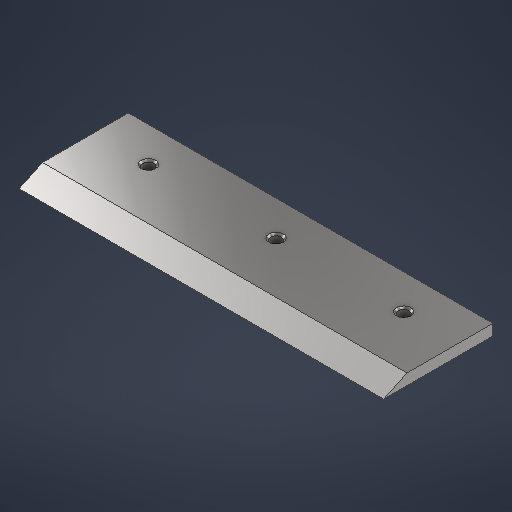
# Autodesk Inventor part: Knife
Saved by Autodesk Inventor 2026.2 (Build 302298010, 298A)
## iProperties
Created: 2026-04-01
Part Number: Knife
Material: Ocel, uhlík
Document SubType Name: Modeling
Designer: zak
Density: 7.85 g/cm^3
Appearance: Pololeštěná
Author: zak
Autodesk Inventor part; units mm, degrees
ref_plane "YZ Plane" through (0, 0, 0) normal (1, 0, 0) x (0, 1, 0)
ref_plane "XZ Plane" through (0, 0, 0) normal (0, 1, 0) x (-1, 0, 0)
ref_plane "XY Plane" through (0, 0, 0) normal (0, 0, 1) x (1, 0, 0)
sketch "Náčrt1" plane through (0, 0, 0) normal (1, 0, 0) x (0, 1, 0)
  line L0 (1.5, 15) -> (-1.5, 15)
  line L1 (-1.5, 15) -> (-1.5, -15)
  line L2 (-1.5, -15) -> (1.5, -15)
  line L3 (1.5, -15) -> (1.5, 15)
  line L4 (1.5, 15) -> (-1.5, -15) construction
  line L5 (-1.5, 15) -> (1.5, -15) construction
  line L6 (-1.5, 15) -> (1.5, 8.5665)
  point P0 (0, 0)
  dimension "d0" = 3
  dimension "d1" = 30
  dimension "d2" = 25
  constraints: 14 end point, 2 midpoint, 2 parallel, 1 horizontal, 1 perpendicular, 1 point on line
  measures "d0" distance between parallel lines of L1 L3
  measures "d1" distance between parallel lines of L0 L2
  measures "d2" angle of L1 L6
extrude "Vysunutí1" add sketch "Náčrt1" along normal mid plane 100 contours L6 L3 L2 L1
sketch "Náčrt2" plane through (-50, -1.5, -15) normal (0, -1, 0) x (1, 0, 0)
  circle A0 centre (85, 9.5) radius 1.5
  circle A1 centre (50, 9.5) radius 1.5
  circle A2 centre (15, 9.5) radius 1.5
  line L0 (0, 0) -> (100, 0) projected
  line L1 (100, 30) -> (100, 0) projected
  line L2 (0, 30) -> (100, 30) projected
  line L3 (0, 0) -> (0, 30) projected
  line L4 (100, 9.5) -> (0, 9.5) construction
  line L5 (50, 0) -> (50, 30) construction
  point P0 (50, 15)
  point P1 (50, 9.5)
  dimension "d5" = 9.5
  dimension "d6" = 3
  dimension "d7" = 35
  dimension "d8" = 3
  constraints: 4 end point, 4 point on line, 3 centre point, 3 midpoint, 1 coincident, 1 perpendicular, 1 other
  measures "d5" distance between parallel lines of L0 L4
  measures "d6" diameter of A1
  measures "d7" distance of A1.centre A2.centre
  measures "d8" diameter of A2
extrude "Vysunutí2" cut sketch "Náčrt2" against normal through all contours A0 | A1 | A2
thread "Závit1" size "M3x0.5" class "6H" standard "ANSI Metric M Profile" full length
thread "Závit2" size "M3x0.5" class "6H" standard "ANSI Metric M Profile" full length
thread "Závit3" size "M3x0.5" class "6H" standard "ANSI Metric M Profile" full length
sketch "Náčrt3" plane through (-50, -1.5, -15) normal (0, -1, 0) x (1, 0, 0)
  circle A0 centre (15, 9.5) radius 1.5 projected
  circle A1 centre (50, 9.5) radius 1.5 projected
  circle A2 centre (85, 9.5) radius 1.5 projected
  line L0 (0, 0) -> (100, 0) projected
  line L1 (100, 30) -> (100, 0) projected
  line L2 (0, 30) -> (100, 30) projected
  line L3 (0, 0) -> (0, 30) projected
  line L4 (99.3391, 0.6963) -> (54.869, 0.6963) construction
  line L5 (54.869, 0.6963) -> (54.869, 9.6594) construction
  line L6 (54.869, 9.6594) -> (99.3391, 9.6594) construction
  line L7 (99.3391, 9.6594) -> (99.3391, 0.6963) construction
  line L8 (98.3181, 1.9686) -> (98.5044, 1.9686)
  line L9 (98.5044, 1.9686) -> (99.0575, 0.8908)
  line L10 (99.0575, 0.8908) -> (99.0575, 1.9686)
  line L11 (99.0575, 1.9686) -> (99.2125, 1.9686)
  line L12 (99.2125, 1.9686) -> (99.2125, 0.7186)
  line L13 (99.2125, 0.7186) -> (98.9765, 0.7186)
  line L14 (98.9765, 0.7186) -> (98.473, 1.7083)
  line L15 (98.473, 1.7083) -> (98.473, 0.7186)
  line L16 (98.473, 0.7186) -> (98.3181, 0.7186)
  line L17 (98.3181, 0.7186) -> (98.3181, 1.9686)
  spline S0 degree 2 poles (97.6698, 1.9899) (97.8946, 1.9899) (98.1418, 1.7376) (98.1418, 1.5046) knots 0 0 0 1 2 2 2
  spline S1 degree 2 poles (98.1418, 1.5046) (98.1418, 1.2757) (97.9017, 1.0042) (97.7083, 1.0042) knots 0 0 0 1 2 2 2
  spline S2 degree 2 poles (97.7083, 1.0042) (97.6211, 1.0042) (97.4864, 1.0549) (97.4368, 1.1086) knots 0 0 0 1 2 2 2
  spline S3 degree 2 poles (97.4368, 1.1086) (97.3861, 1.1623) (97.3324, 1.3172) (97.3324, 1.4297) knots 0 0 0 1 2 2 2
  line L18 (97.3324, 1.4297) -> (97.3324, 1.5158)
  line L19 (97.3324, 1.5158) -> (97.9818, 1.5158)
  spline S4 degree 2 poles (97.9818, 1.5158) (97.9818, 1.6789) (97.8177, 1.8521) (97.6718, 1.8521) knots 0 0 0 1 2 2 2
  spline S5 degree 2 poles (97.6718, 1.8521) (97.6201, 1.8521) (97.5198, 1.8288) (97.4793, 1.8106) knots 0 0 0 1 2 2 2
  spline S6 degree 2 poles (97.4793, 1.8106) (97.4368, 1.7903) (97.378, 1.7548) (97.3588, 1.7386) knots 0 0 0 1 2 2 2
  line L20 (97.3588, 1.7386) -> (97.3497, 1.7386)
  line L21 (97.3497, 1.7386) -> (97.3497, 1.9108)
  spline S7 degree 2 poles (97.3497, 1.9108) (97.377, 1.922) (97.4601, 1.9544) (97.4925, 1.9635) knots 0 0 0 1 2 2 2
  spline S8 degree 2 poles (97.4925, 1.9635) (97.5381, 1.9767) (97.613, 1.9899) (97.6698, 1.9899) knots 0 0 0 1 2 2 2
  spline S9 degree 2 poles (97.4864, 1.3952) (97.4884, 1.3314) (97.5148, 1.2382) (97.5401, 1.2068) knots 0 0 0 1 2 2 2
  spline S10 degree 2 poles (97.5401, 1.2068) (97.5674, 1.1714) (97.6536, 1.1339) (97.7174, 1.1339) knots 0 0 0 1 2 2 2
  spline S11 degree 2 poles (97.7174, 1.1339) (97.7802, 1.1339) (97.8683, 1.1714) (97.9048, 1.2078) knots 0 0 0 1 2 2 2
  spline S12 degree 2 poles (97.9048, 1.2078) (97.9402, 1.2453) (97.9767, 1.3355) (97.9818, 1.3952) knots 0 0 0 1 2 2 2
  line L22 (97.9818, 1.3952) -> (97.4864, 1.3952)
  spline S13 degree 2 poles (96.4015, 1.4996) (96.4015, 1.7366) (96.6294, 1.9949) (96.8199, 1.9949) knots 0 0 0 1 2 2 2
  spline S14 degree 2 poles (96.8199, 1.9949) (97.0154, 1.9949) (97.2392, 1.7285) (97.2392, 1.4996) knots 0 0 0 1 2 2 2
  spline S15 degree 2 poles (97.2392, 1.4996) (97.2392, 1.2646) (97.0083, 1.0042) (96.8199, 1.0042) knots 0 0 0 1 2 2 2
  spline S16 degree 2 poles (96.8199, 1.0042) (96.6294, 1.0042) (96.4015, 1.2636) (96.4015, 1.4996) knots 0 0 0 1 2 2 2
  spline S17 degree 2 poles (96.5646, 1.4996) (96.5646, 1.3172) (96.6973, 1.14) (96.8199, 1.14) knots 0 0 0 1 2 2 2
  spline S18 degree 2 poles (96.8199, 1.14) (96.9424, 1.14) (97.0762, 1.3172) (97.0762, 1.4996) knots 0 0 0 1 2 2 2
  spline S19 degree 2 poles (97.0762, 1.4996) (97.0762, 1.6768) (96.9424, 1.8592) (96.8199, 1.8592) knots 0 0 0 1 2 2 2
  spline S20 degree 2 poles (96.8199, 1.8592) (96.6983, 1.8592) (96.5646, 1.6799) (96.5646, 1.4996) knots 0 0 0 1 2 2 2
  spline S21 degree 2 poles (95.8788, 1.9909) (96.0146, 1.9909) (96.205, 1.9341) (96.2891, 1.8936) knots 0 0 0 1 2 2 2
  line L23 (96.2891, 1.8936) -> (96.2891, 1.685)
  line L24 (96.2891, 1.685) -> (96.2769, 1.685)
  spline S22 degree 2 poles (96.2769, 1.685) (96.1949, 1.7619) (95.9872, 1.847) (95.891, 1.847) knots 0 0 0 1 2 2 2
  spline S23 degree 2 poles (95.891, 1.847) (95.7532, 1.847) (95.6124, 1.7326) (95.6124, 1.6384) knots 0 0 0 1 2 2 2
  spline S24 degree 2 poles (95.6124, 1.6384) (95.6124, 1.5634) (95.6864, 1.4702) (95.7664, 1.4469) knots 0 0 0 1 2 2 2
  spline S25 degree 2 poles (95.7664, 1.4469) (95.8241, 1.4307) (95.9204, 1.4084) (95.9923, 1.3902) knots 0 0 0 1 2 2 2
  spline S26 degree 2 poles (95.9923, 1.3902) (96.0571, 1.373) (96.1594, 1.3213) (96.1989, 1.2798) knots 0 0 0 1 2 2 2
  spline S27 degree 2 poles (96.1989, 1.2798) (96.2374, 1.2382) (96.28, 1.1268) (96.28, 1.0539) knots 0 0 0 1 2 2 2
  spline S28 degree 2 poles (96.28, 1.0539) (96.28, 0.9019) (96.0429, 0.6963) (95.8596, 0.6963) knots 0 0 0 1 2 2 2
  spline S29 degree 2 poles (95.8596, 0.6963) (95.7542, 0.6963) (95.5679, 0.7378) (95.4878, 0.7773) knots 0 0 0 1 2 2 2
  line L25 (95.4878, 0.7773) -> (95.4878, 0.9759)
  line L26 (95.4878, 0.9759) -> (95.5, 0.9759)
  spline S30 degree 2 poles (95.5, 0.9759) (95.5598, 0.9212) (95.7461, 0.8401) (95.8484, 0.8401) knots 0 0 0 1 2 2 2
  spline S31 degree 2 poles (95.8484, 0.8401) (95.9639, 0.8401) (96.1068, 0.9485) (96.1068, 1.0367) knots 0 0 0 1 2 2 2
  spline S32 degree 2 poles (96.1068, 1.0367) (96.1068, 1.1157) (96.0227, 1.2099) (95.9437, 1.2311) knots 0 0 0 1 2 2 2
  spline S33 degree 2 poles (95.9437, 1.2311) (95.891, 1.2453) (95.738, 1.2818) (95.6874, 1.297) knots 0 0 0 1 2 2 2
  spline S34 degree 2 poles (95.6874, 1.297) (95.5587, 1.3365) (95.4392, 1.4955) (95.4392, 1.612) knots 0 0 0 1 2 2 2
  spline S35 degree 2 poles (95.4392, 1.612) (95.4392, 1.686) (95.499, 1.8278) (95.5527, 1.8774) knots 0 0 0 1 2 2 2
  spline S36 degree 2 poles (95.5527, 1.8774) (95.6124, 1.9321) (95.7644, 1.9909) (95.8788, 1.9909) knots 0 0 0 1 2 2 2
  line L27 (94.5529, 1.9686) -> (94.7109, 1.9686)
  line L28 (94.7109, 1.9686) -> (94.7109, 1.8653)
  spline S37 degree 2 poles (94.7109, 1.8653) (94.7838, 1.9291) (94.9145, 1.9949) (94.9955, 1.9949) knots 0 0 0 1 2 2 2
  spline S38 degree 2 poles (94.9955, 1.9949) (95.0563, 1.9949) (95.1647, 1.9544) (95.2042, 1.9108) knots 0 0 0 1 2 2 2
  spline S39 degree 2 poles (95.2042, 1.9108) (95.2447, 1.8673) (95.2893, 1.7346) (95.2893, 1.6394) knots 0 0 0 1 2 2 2
  line L29 (95.2893, 1.6394) -> (95.2893, 1.0306)
  line L30 (95.2893, 1.0306) -> (95.1313, 1.0306)
  line L31 (95.1313, 1.0306) -> (95.1313, 1.5654)
  spline S40 degree 2 poles (95.1313, 1.5654) (95.1313, 1.6404) (95.1201, 1.7386) (95.1009, 1.7751) knots 0 0 0 1 2 2 2
  spline S41 degree 2 poles (95.1009, 1.7751) (95.0816, 1.8116) (95.0158, 1.845) (94.954, 1.845) knots 0 0 0 1 2 2 2
  spline S42 degree 2 poles (94.954, 1.845) (94.8963, 1.845) (94.7656, 1.7792) (94.7109, 1.7315) knots 0 0 0 1 2 2 2
  line L32 (94.7109, 1.7315) -> (94.7109, 1.0306)
  line L33 (94.7109, 1.0306) -> (94.5529, 1.0306)
  line L34 (94.5529, 1.0306) -> (94.5529, 1.9686)
  line L35 (93.2603, 1.9686) -> (93.2603, 1.4256)
  spline S43 degree 2 poles (93.2603, 1.4256) (93.2603, 1.3608) (93.2704, 1.2504) (93.2867, 1.22) knots 0 0 0 1 2 2 2
  spline S44 degree 2 poles (93.2867, 1.22) (93.3029, 1.1866) (93.3647, 1.1542) (93.4183, 1.1542) knots 0 0 0 1 2 2 2
  spline S45 degree 2 poles (93.4183, 1.1542) (93.467, 1.1542) (93.5784, 1.2139) (93.6371, 1.2707) knots 0 0 0 1 2 2 2
  spline S46 degree 2 poles (93.6371, 1.2707) (93.6361, 1.2848) (93.6341, 1.3243) (93.6341, 1.3507) knots 0 0 0 1 2 2 2
  line L36 (93.6341, 1.3507) -> (93.6341, 1.9686)
  line L37 (93.6341, 1.9686) -> (93.7921, 1.9686)
  line L38 (93.7921, 1.9686) -> (93.7921, 1.4256)
  spline S47 degree 2 poles (93.7921, 1.4256) (93.7921, 1.3608) (93.8023, 1.2504) (93.8185, 1.22) knots 0 0 0 1 2 2 2
  spline S48 degree 2 poles (93.8185, 1.22) (93.8347, 1.1866) (93.8965, 1.1542) (93.9501, 1.1542) knots 0 0 0 1 2 2 2
  spline S49 degree 2 poles (93.9501, 1.1542) (94.0008, 1.1542) (94.1132, 1.218) (94.1659, 1.2676) knots 0 0 0 1 2 2 2
  line L39 (94.1659, 1.2676) -> (94.1659, 1.9686)
  line L40 (94.1659, 1.9686) -> (94.3239, 1.9686)
  line L41 (94.3239, 1.9686) -> (94.3239, 1.0306)
  line L42 (94.3239, 1.0306) -> (94.1659, 1.0306)
  line L43 (94.1659, 1.0306) -> (94.1659, 1.1339)
  spline S50 degree 2 poles (94.1659, 1.1339) (94.1041, 1.0721) (93.9826, 1.0042) (93.9096, 1.0042) knots 0 0 0 1 2 2 2
  spline S51 degree 2 poles (93.9096, 1.0042) (93.8266, 1.0042) (93.6979, 1.0802) (93.6645, 1.1663) knots 0 0 0 1 2 2 2
  spline S52 degree 2 poles (93.6645, 1.1663) (93.5926, 1.0863) (93.4568, 1.0042) (93.3778, 1.0042) knots 0 0 0 1 2 2 2
  spline S53 degree 2 poles (93.3778, 1.0042) (93.317, 1.0042) (93.2178, 1.0417) (93.1813, 1.0843) knots 0 0 0 1 2 2 2
  spline S54 degree 2 poles (93.1813, 1.0843) (93.1438, 1.1268) (93.1023, 1.2544) (93.1023, 1.3507) knots 0 0 0 1 2 2 2
  line L44 (93.1023, 1.3507) -> (93.1023, 1.9686)
  line L45 (93.1023, 1.9686) -> (93.2603, 1.9686)
  spline S55 degree 2 poles (92.4732, 1.9899) (92.6981, 1.9899) (92.9453, 1.7376) (92.9453, 1.5046) knots 0 0 0 1 2 2 2
  spline S56 degree 2 poles (92.9453, 1.5046) (92.9453, 1.2757) (92.7052, 1.0042) (92.5117, 1.0042) knots 0 0 0 1 2 2 2
  spline S57 degree 2 poles (92.5117, 1.0042) (92.4246, 1.0042) (92.2899, 1.0549) (92.2403, 1.1086) knots 0 0 0 1 2 2 2
  spline S58 degree 2 poles (92.2403, 1.1086) (92.1896, 1.1623) (92.1359, 1.3172) (92.1359, 1.4297) knots 0 0 0 1 2 2 2
  line L46 (92.1359, 1.4297) -> (92.1359, 1.5158)
  line L47 (92.1359, 1.5158) -> (92.7852, 1.5158)
  spline S59 degree 2 poles (92.7852, 1.5158) (92.7852, 1.6789) (92.6211, 1.8521) (92.4753, 1.8521) knots 0 0 0 1 2 2 2
  spline S60 degree 2 poles (92.4753, 1.8521) (92.4236, 1.8521) (92.3233, 1.8288) (92.2828, 1.8106) knots 0 0 0 1 2 2 2
  spline S61 degree 2 poles (92.2828, 1.8106) (92.2403, 1.7903) (92.1815, 1.7548) (92.1623, 1.7386) knots 0 0 0 1 2 2 2
  line L48 (92.1623, 1.7386) -> (92.1531, 1.7386)
  line L49 (92.1531, 1.7386) -> (92.1531, 1.9108)
  spline S62 degree 2 poles (92.1531, 1.9108) (92.1805, 1.922) (92.2636, 1.9544) (92.296, 1.9635) knots 0 0 0 1 2 2 2
  spline S63 degree 2 poles (92.296, 1.9635) (92.3416, 1.9767) (92.4165, 1.9899) (92.4732, 1.9899) knots 0 0 0 1 2 2 2
  spline S64 degree 2 poles (92.2899, 1.3952) (92.2919, 1.3314) (92.3183, 1.2382) (92.3436, 1.2068) knots 0 0 0 1 2 2 2
  spline S65 degree 2 poles (92.3436, 1.2068) (92.3709, 1.1714) (92.457, 1.1339) (92.5209, 1.1339) knots 0 0 0 1 2 2 2
  spline S66 degree 2 poles (92.5209, 1.1339) (92.5837, 1.1339) (92.6718, 1.1714) (92.7083, 1.2078) knots 0 0 0 1 2 2 2
  spline S67 degree 2 poles (92.7083, 1.2078) (92.7437, 1.2453) (92.7802, 1.3355) (92.7852, 1.3952) knots 0 0 0 1 2 2 2
  line L50 (92.7852, 1.3952) -> (92.2899, 1.3952)
  spline S68 degree 2 poles (91.6031, 1.9899) (91.7004, 1.9899) (91.8614, 1.9301) (91.9192, 1.8693) knots 0 0 0 1 2 2 2
  spline S69 degree 2 poles (91.9192, 1.8693) (91.9769, 1.8095) (92.0407, 1.6252) (92.0407, 1.5016) knots 0 0 0 1 2 2 2
  spline S70 degree 2 poles (92.0407, 1.5016) (92.0407, 1.378) (91.9749, 1.1977) (91.9192, 1.1369) knots 0 0 0 1 2 2 2
  spline S71 degree 2 poles (91.9192, 1.1369) (91.8634, 1.0751) (91.6983, 1.0093) (91.6031, 1.0093) knots 0 0 0 1 2 2 2
  spline S72 degree 2 poles (91.6031, 1.0093) (91.5261, 1.0093) (91.3823, 1.0529) (91.3266, 1.0812) knots 0 0 0 1 2 2 2
  line L51 (91.3266, 1.0812) -> (91.3266, 1.2585)
  line L52 (91.3266, 1.2585) -> (91.3357, 1.2585)
  spline S73 degree 2 poles (91.3357, 1.2585) (91.3529, 1.2443) (91.4056, 1.2078) (91.4431, 1.1886) knots 0 0 0 1 2 2 2
  spline S74 degree 2 poles (91.4431, 1.1886) (91.4765, 1.1724) (91.5656, 1.1471) (91.6061, 1.1471) knots 0 0 0 1 2 2 2
  spline S75 degree 2 poles (91.6061, 1.1471) (91.7287, 1.1471) (91.8776, 1.3324) (91.8776, 1.5016) knots 0 0 0 1 2 2 2
  spline S76 degree 2 poles (91.8776, 1.5016) (91.8776, 1.6667) (91.7338, 1.8521) (91.6061, 1.8521) knots 0 0 0 1 2 2 2
  spline S77 degree 2 poles (91.6061, 1.8521) (91.5292, 1.8521) (91.3894, 1.7883) (91.3357, 1.7386) knots 0 0 0 1 2 2 2
  line L53 (91.3357, 1.7386) -> (91.3266, 1.7386)
  line L54 (91.3266, 1.7386) -> (91.3266, 1.9159)
  spline S78 degree 2 poles (91.3266, 1.9159) (91.3499, 1.9271) (91.4208, 1.9585) (91.4491, 1.9655) knots 0 0 0 1 2 2 2
  spline S79 degree 2 poles (91.4491, 1.9655) (91.4897, 1.9777) (91.5535, 1.9899) (91.6031, 1.9899) knots 0 0 0 1 2 2 2
  line L55 (98.1408, 4.0267) -> (98.3069, 4.0267)
  line L56 (98.3069, 4.0267) -> (98.3069, 2.9499)
  line L57 (98.3069, 2.9499) -> (98.6331, 3.6823)
  line L58 (98.6331, 3.6823) -> (98.7344, 3.6823)
  line L59 (98.7344, 3.6823) -> (99.0575, 2.9499)
  line L60 (99.0575, 2.9499) -> (99.0575, 4.0267)
  line L61 (99.0575, 4.0267) -> (99.2125, 4.0267)
  line L62 (99.2125, 4.0267) -> (99.2125, 2.7767)
  line L63 (99.2125, 2.7767) -> (98.9856, 2.7767)
  line L64 (98.9856, 2.7767) -> (98.6736, 3.4726)
  line L65 (98.6736, 3.4726) -> (98.3717, 2.7767)
  line L66 (98.3717, 2.7767) -> (98.1408, 2.7767)
  line L67 (98.1408, 2.7767) -> (98.1408, 4.0267)
  spline S80 degree 2 poles (97.377, 3.9274) (97.3963, 3.9416) (97.4611, 3.9922) (97.4915, 4.0074) knots 0 0 0 1 2 2 2
  spline S81 degree 2 poles (97.4915, 4.0074) (97.533, 4.0297) (97.611, 4.053) (97.6819, 4.053) knots 0 0 0 1 2 2 2
  spline S82 degree 2 poles (97.6819, 4.053) (97.7397, 4.053) (97.844, 4.0095) (97.8835, 3.9699) knots 0 0 0 1 2 2 2
  spline S83 degree 2 poles (97.8835, 3.9699) (97.921, 3.9315) (97.9666, 3.818) (97.9666, 3.7552) knots 0 0 0 1 2 2 2
  spline S84 degree 2 poles (97.9666, 3.7552) (97.9666, 3.658) (97.8845, 3.5202) (97.7954, 3.4807) knots 0 0 0 1 2 2 2
  spline S85 degree 2 poles (97.7954, 3.4807) (97.7164, 3.4442) (97.5016, 3.4169) (97.377, 3.4098) knots 0 0 0 1 2 2 2
  line L68 (97.377, 3.4098) -> (97.377, 3.3794)
  spline S86 degree 2 poles (97.377, 3.3794) (97.377, 3.3247) (97.4104, 3.2568) (97.4408, 3.2376) knots 0 0 0 1 2 2 2
  spline S87 degree 2 poles (97.4408, 3.2376) (97.4712, 3.2183) (97.5583, 3.2062) (97.6049, 3.2062) knots 0 0 0 1 2 2 2
  spline S88 degree 2 poles (97.6049, 3.2062) (97.6596, 3.2062) (97.8075, 3.2386) (97.8815, 3.27) knots 0 0 0 1 2 2 2
  line L69 (97.8815, 3.27) -> (97.8906, 3.27)
  line L70 (97.8906, 3.27) -> (97.8906, 3.1089)
  spline S89 degree 2 poles (97.8906, 3.1089) (97.847, 3.0968) (97.6839, 3.0664) (97.6039, 3.0664) knots 0 0 0 1 2 2 2
  spline S90 degree 2 poles (97.6039, 3.0664) (97.5067, 3.0664) (97.374, 3.0968) (97.3213, 3.1363) knots 0 0 0 1 2 2 2
  spline S91 degree 2 poles (97.3213, 3.1363) (97.2696, 3.1748) (97.219, 3.2973) (97.219, 3.3855) knots 0 0 0 1 2 2 2
  line L71 (97.219, 3.3855) -> (97.219, 4.0267)
  line L72 (97.219, 4.0267) -> (97.377, 4.0267)
  line L73 (97.377, 4.0267) -> (97.377, 3.9274)
  line L74 (97.377, 3.7957) -> (97.377, 3.5354)
  spline S92 degree 2 poles (97.377, 3.5354) (97.4337, 3.5405) (97.6049, 3.5577) (97.6586, 3.5739) knots 0 0 0 1 2 2 2
  spline S93 degree 2 poles (97.6586, 3.5739) (97.7214, 3.5931) (97.8035, 3.6732) (97.8035, 3.7441) knots 0 0 0 1 2 2 2
  spline S94 degree 2 poles (97.8035, 3.7441) (97.8035, 3.8251) (97.7123, 3.9071) (97.6252, 3.9071) knots 0 0 0 1 2 2 2
  spline S95 degree 2 poles (97.6252, 3.9071) (97.5512, 3.9071) (97.4297, 3.8433) (97.377, 3.7957) knots 0 0 0 1 2 2 2
  line L75 (96.2759, 4.0267) -> (96.4339, 4.0267)
  line L76 (96.4339, 4.0267) -> (96.4339, 3.9315)
  spline S96 degree 2 poles (96.4339, 3.9315) (96.4704, 3.9618) (96.5241, 4.0024) (96.5606, 4.0196) knots 0 0 0 1 2 2 2
  spline S97 degree 2 poles (96.5606, 4.0196) (96.594, 4.0358) (96.6659, 4.053) (96.7135, 4.053) knots 0 0 0 1 2 2 2
  spline S98 degree 2 poles (96.7135, 4.053) (96.7905, 4.053) (96.9202, 3.9892) (96.9657, 3.9274) knots 0 0 0 1 2 2 2
  spline S99 degree 2 poles (96.9657, 3.9274) (97.0113, 3.8656) (97.062, 3.6833) (97.062, 3.5648) knots 0 0 0 1 2 2 2
  spline S100 degree 2 poles (97.062, 3.5648) (97.062, 3.4412) (96.9982, 3.2609) (96.9424, 3.193) knots 0 0 0 1 2 2 2
  spline S101 degree 2 poles (96.9424, 3.193) (96.8908, 3.1322) (96.7459, 3.0623) (96.6659, 3.0623) knots 0 0 0 1 2 2 2
  spline S102 degree 2 poles (96.6659, 3.0623) (96.596, 3.0623) (96.4917, 3.0937) (96.4339, 3.1261) knots 0 0 0 1 2 2 2
  line L77 (96.4339, 3.1261) -> (96.4339, 2.721)
  line L78 (96.4339, 2.721) -> (96.2759, 2.721)
  line L79 (96.2759, 2.721) -> (96.2759, 4.0267)
  line L80 (96.4339, 3.7988) -> (96.4339, 3.2568)
  spline S103 degree 2 poles (96.4339, 3.2568) (96.4927, 3.2285) (96.5859, 3.2072) (96.6396, 3.2072) knots 0 0 0 1 2 2 2
  spline S104 degree 2 poles (96.6396, 3.2072) (96.7611, 3.2072) (96.8989, 3.3895) (96.8989, 3.5617) knots 0 0 0 1 2 2 2
  spline S105 degree 2 poles (96.8989, 3.5617) (96.8989, 3.7279) (96.7935, 3.9031) (96.6771, 3.9031) knots 0 0 0 1 2 2 2
  spline S106 degree 2 poles (96.6771, 3.9031) (96.6153, 3.9031) (96.4897, 3.8464) (96.4339, 3.7988) knots 0 0 0 1 2 2 2
  spline S107 degree 2 poles (95.6398, 4.0479) (95.8647, 4.0479) (96.1118, 3.7957) (96.1118, 3.5627) knots 0 0 0 1 2 2 2
  spline S108 degree 2 poles (96.1118, 3.5627) (96.1118, 3.3338) (95.8717, 3.0623) (95.6783, 3.0623) knots 0 0 0 1 2 2 2
  spline S109 degree 2 poles (95.6783, 3.0623) (95.5912, 3.0623) (95.4564, 3.113) (95.4068, 3.1667) knots 0 0 0 1 2 2 2
  spline S110 degree 2 poles (95.4068, 3.1667) (95.3561, 3.2204) (95.3025, 3.3753) (95.3025, 3.4878) knots 0 0 0 1 2 2 2
  line L81 (95.3025, 3.4878) -> (95.3025, 3.5739)
  line L82 (95.3025, 3.5739) -> (95.9518, 3.5739)
  spline S111 degree 2 poles (95.9518, 3.5739) (95.9518, 3.737) (95.7877, 3.9102) (95.6418, 3.9102) knots 0 0 0 1 2 2 2
  spline S112 degree 2 poles (95.6418, 3.9102) (95.5901, 3.9102) (95.4899, 3.8869) (95.4493, 3.8687) knots 0 0 0 1 2 2 2
  spline S113 degree 2 poles (95.4493, 3.8687) (95.4068, 3.8484) (95.348, 3.8129) (95.3288, 3.7967) knots 0 0 0 1 2 2 2
  line L83 (95.3288, 3.7967) -> (95.3197, 3.7967)
  line L84 (95.3197, 3.7967) -> (95.3197, 3.9689)
  spline S114 degree 2 poles (95.3197, 3.9689) (95.347, 3.9801) (95.4301, 4.0125) (95.4625, 4.0216) knots 0 0 0 1 2 2 2
  spline S115 degree 2 poles (95.4625, 4.0216) (95.5081, 4.0348) (95.583, 4.0479) (95.6398, 4.0479) knots 0 0 0 1 2 2 2
  spline S116 degree 2 poles (95.4564, 3.4533) (95.4585, 3.3895) (95.4848, 3.2963) (95.5101, 3.2649) knots 0 0 0 1 2 2 2
  spline S117 degree 2 poles (95.5101, 3.2649) (95.5375, 3.2295) (95.6236, 3.192) (95.6874, 3.192) knots 0 0 0 1 2 2 2
  spline S118 degree 2 poles (95.6874, 3.192) (95.7502, 3.192) (95.8383, 3.2295) (95.8748, 3.2659) knots 0 0 0 1 2 2 2
  spline S119 degree 2 poles (95.8748, 3.2659) (95.9102, 3.3034) (95.9467, 3.3936) (95.9518, 3.4533) knots 0 0 0 1 2 2 2
  line L85 (95.9518, 3.4533) -> (95.4564, 3.4533)
  spline S120 degree 2 poles (93.8195, 3.5425) (93.8195, 3.7724) (94.0423, 4.053) (94.2105, 4.053) knots 0 0 0 1 2 2 2
  spline S121 degree 2 poles (94.2105, 4.053) (94.2865, 4.053) (94.3948, 4.0155) (94.4475, 3.9831) knots 0 0 0 1 2 2 2
  line L86 (94.4475, 3.9831) -> (94.4576, 4.0267)
  line L87 (94.4576, 4.0267) -> (94.6055, 4.0267)
  line L88 (94.6055, 4.0267) -> (94.6055, 2.721)
  line L89 (94.6055, 2.721) -> (94.4475, 2.721)
  line L90 (94.4475, 2.721) -> (94.4475, 3.1869)
  spline S122 degree 2 poles (94.4475, 3.1869) (94.3877, 3.1332) (94.249, 3.0623) (94.1608, 3.0623) knots 0 0 0 1 2 2 2
  spline S123 degree 2 poles (94.1608, 3.0623) (94.0018, 3.0623) (93.8195, 3.3166) (93.8195, 3.5425) knots 0 0 0 1 2 2 2
  spline S124 degree 2 poles (93.9826, 3.5546) (93.9826, 3.3865) (94.0849, 3.2123) (94.1983, 3.2123) knots 0 0 0 1 2 2 2
  spline S125 degree 2 poles (94.1983, 3.2123) (94.2621, 3.2123) (94.3938, 3.273) (94.4475, 3.3196) knots 0 0 0 1 2 2 2
  line L91 (94.4475, 3.3196) -> (94.4475, 3.8575)
  spline S126 degree 2 poles (94.4475, 3.8575) (94.3877, 3.8869) (94.2956, 3.9112) (94.2409, 3.9112) knots 0 0 0 1 2 2 2
  spline S127 degree 2 poles (94.2409, 3.9112) (94.1203, 3.9112) (93.9826, 3.74) (93.9826, 3.5546) knots 0 0 0 1 2 2 2
  line L92 (92.9189, 3.0887) -> (93.4234, 4.3721)
  line L93 (93.4234, 4.3721) -> (93.5926, 4.3721)
  line L94 (93.5926, 4.3721) -> (93.4244, 3.9811)
  line L95 (93.4244, 3.9811) -> (93.7648, 3.0887)
  line L96 (93.7648, 3.0887) -> (93.5946, 3.0887)
  line L97 (93.5946, 3.0887) -> (93.3383, 3.7836)
  line L98 (93.3383, 3.7836) -> (93.083, 3.0887)
  line L99 (93.083, 3.0887) -> (92.9189, 3.0887)
  line L100 (91.3438, 2.7767) -> (91.7743, 4.0267)
  line L101 (91.7743, 4.0267) -> (91.9536, 4.0267)
  line L102 (91.9536, 4.0267) -> (92.3841, 2.7767)
  line L103 (92.3841, 2.7767) -> (92.2058, 2.7767)
  line L104 (92.2058, 2.7767) -> (91.8594, 3.815)
  line L105 (91.8594, 3.815) -> (91.513, 2.7767)
  line L106 (91.513, 2.7767) -> (91.3438, 2.7767)
  spline S128 degree 2 poles (90.7137, 3.9274) (90.733, 3.9416) (90.7978, 3.9922) (90.8282, 4.0074) knots 0 0 0 1 2 2 2
  spline S129 degree 2 poles (90.8282, 4.0074) (90.8697, 4.0297) (90.9477, 4.053) (91.0186, 4.053) knots 0 0 0 1 2 2 2
  spline S130 degree 2 poles (91.0186, 4.053) (91.0764, 4.053) (91.1807, 4.0095) (91.2202, 3.9699) knots 0 0 0 1 2 2 2
  spline S131 degree 2 poles (91.2202, 3.9699) (91.2577, 3.9315) (91.3033, 3.818) (91.3033, 3.7552) knots 0 0 0 1 2 2 2
  spline S132 degree 2 poles (91.3033, 3.7552) (91.3033, 3.658) (91.2212, 3.5202) (91.1321, 3.4807) knots 0 0 0 1 2 2 2
  spline S133 degree 2 poles (91.1321, 3.4807) (91.0531, 3.4442) (90.8383, 3.4169) (90.7137, 3.4098) knots 0 0 0 1 2 2 2
  line L107 (90.7137, 3.4098) -> (90.7137, 3.3794)
  spline S134 degree 2 poles (90.7137, 3.3794) (90.7137, 3.3247) (90.7472, 3.2568) (90.7775, 3.2376) knots 0 0 0 1 2 2 2
  spline S135 degree 2 poles (90.7775, 3.2376) (90.8079, 3.2183) (90.895, 3.2062) (90.9416, 3.2062) knots 0 0 0 1 2 2 2
  spline S136 degree 2 poles (90.9416, 3.2062) (90.9963, 3.2062) (91.1442, 3.2386) (91.2182, 3.27) knots 0 0 0 1 2 2 2
  line L108 (91.2182, 3.27) -> (91.2273, 3.27)
  line L109 (91.2273, 3.27) -> (91.2273, 3.1089)
  spline S137 degree 2 poles (91.2273, 3.1089) (91.1837, 3.0968) (91.0207, 3.0664) (90.9406, 3.0664) knots 0 0 0 1 2 2 2
  spline S138 degree 2 poles (90.9406, 3.0664) (90.8434, 3.0664) (90.7107, 3.0968) (90.658, 3.1363) knots 0 0 0 1 2 2 2
  spline S139 degree 2 poles (90.658, 3.1363) (90.6063, 3.1748) (90.5557, 3.2973) (90.5557, 3.3855) knots 0 0 0 1 2 2 2
  line L110 (90.5557, 3.3855) -> (90.5557, 4.0267)
  line L111 (90.5557, 4.0267) -> (90.7137, 4.0267)
  line L112 (90.7137, 4.0267) -> (90.7137, 3.9274)
  line L113 (90.7137, 3.7957) -> (90.7137, 3.5354)
  spline S140 degree 2 poles (90.7137, 3.5354) (90.7704, 3.5405) (90.9416, 3.5577) (90.9953, 3.5739) knots 0 0 0 1 2 2 2
  spline S141 degree 2 poles (90.9953, 3.5739) (91.0581, 3.5931) (91.1402, 3.6732) (91.1402, 3.7441) knots 0 0 0 1 2 2 2
  spline S142 degree 2 poles (91.1402, 3.7441) (91.1402, 3.8251) (91.049, 3.9071) (90.9619, 3.9071) knots 0 0 0 1 2 2 2
  spline S143 degree 2 poles (90.9619, 3.9071) (90.888, 3.9071) (90.7664, 3.8433) (90.7137, 3.7957) knots 0 0 0 1 2 2 2
  line L114 (89.6126, 4.0267) -> (89.7707, 4.0267)
  line L115 (89.7707, 4.0267) -> (89.7707, 3.9315)
  spline S144 degree 2 poles (89.7707, 3.9315) (89.8071, 3.9618) (89.8608, 4.0024) (89.8973, 4.0196) knots 0 0 0 1 2 2 2
  spline S145 degree 2 poles (89.8973, 4.0196) (89.9307, 4.0358) (90.0026, 4.053) (90.0502, 4.053) knots 0 0 0 1 2 2 2
  spline S146 degree 2 poles (90.0502, 4.053) (90.1272, 4.053) (90.2569, 3.9892) (90.3025, 3.9274) knots 0 0 0 1 2 2 2
  spline S147 degree 2 poles (90.3025, 3.9274) (90.348, 3.8656) (90.3987, 3.6833) (90.3987, 3.5648) knots 0 0 0 1 2 2 2
  spline S148 degree 2 poles (90.3987, 3.5648) (90.3987, 3.4412) (90.3349, 3.2609) (90.2792, 3.193) knots 0 0 0 1 2 2 2
  spline S149 degree 2 poles (90.2792, 3.193) (90.2275, 3.1322) (90.0826, 3.0623) (90.0026, 3.0623) knots 0 0 0 1 2 2 2
  spline S150 degree 2 poles (90.0026, 3.0623) (89.9327, 3.0623) (89.8284, 3.0937) (89.7707, 3.1261) knots 0 0 0 1 2 2 2
  line L116 (89.7707, 3.1261) -> (89.7707, 2.721)
  line L117 (89.7707, 2.721) -> (89.6126, 2.721)
  line L118 (89.6126, 2.721) -> (89.6126, 4.0267)
  line L119 (89.7707, 3.7988) -> (89.7707, 3.2568)
  spline S151 degree 2 poles (89.7707, 3.2568) (89.8294, 3.2285) (89.9226, 3.2072) (89.9763, 3.2072) knots 0 0 0 1 2 2 2
  spline S152 degree 2 poles (89.9763, 3.2072) (90.0978, 3.2072) (90.2356, 3.3895) (90.2356, 3.5617) knots 0 0 0 1 2 2 2
  spline S153 degree 2 poles (90.2356, 3.5617) (90.2356, 3.7279) (90.1303, 3.9031) (90.0138, 3.9031) knots 0 0 0 1 2 2 2
  spline S154 degree 2 poles (90.0138, 3.9031) (89.952, 3.9031) (89.8264, 3.8464) (89.7707, 3.7988) knots 0 0 0 1 2 2 2
  line L120 (89.2226, 4.0267) -> (89.3807, 4.0267)
  line L121 (89.3807, 4.0267) -> (89.3807, 3.0887)
  line L122 (89.3807, 3.0887) -> (89.2226, 3.0887)
  line L123 (89.2226, 3.0887) -> (89.2226, 4.0267)
  line L124 (89.2115, 2.9327) -> (89.3908, 2.9327)
  line L125 (89.3908, 2.9327) -> (89.3908, 2.7686)
  line L126 (89.3908, 2.7686) -> (89.2115, 2.7686)
  line L127 (89.2115, 2.7686) -> (89.2115, 2.9327)
  line L128 (87.9271, 4.0267) -> (87.9271, 3.4837)
  spline S155 degree 2 poles (87.9271, 3.4837) (87.9271, 3.4189) (87.9372, 3.3085) (87.9534, 3.2781) knots 0 0 0 1 2 2 2
  spline S156 degree 2 poles (87.9534, 3.2781) (87.9696, 3.2447) (88.0314, 3.2123) (88.0851, 3.2123) knots 0 0 0 1 2 2 2
  spline S157 degree 2 poles (88.0851, 3.2123) (88.1337, 3.2123) (88.2451, 3.272) (88.3039, 3.3287) knots 0 0 0 1 2 2 2
  spline S158 degree 2 poles (88.3039, 3.3287) (88.3029, 3.3429) (88.3008, 3.3824) (88.3008, 3.4088) knots 0 0 0 1 2 2 2
  line L129 (88.3008, 3.4088) -> (88.3008, 4.0267)
  line L130 (88.3008, 4.0267) -> (88.4589, 4.0267)
  line L131 (88.4589, 4.0267) -> (88.4589, 3.4837)
  spline S159 degree 2 poles (88.4589, 3.4837) (88.4589, 3.4189) (88.469, 3.3085) (88.4852, 3.2781) knots 0 0 0 1 2 2 2
  spline S160 degree 2 poles (88.4852, 3.2781) (88.5014, 3.2447) (88.5632, 3.2123) (88.6169, 3.2123) knots 0 0 0 1 2 2 2
  spline S161 degree 2 poles (88.6169, 3.2123) (88.6675, 3.2123) (88.78, 3.2761) (88.8326, 3.3257) knots 0 0 0 1 2 2 2
  line L132 (88.8326, 3.3257) -> (88.8326, 4.0267)
  line L133 (88.8326, 4.0267) -> (88.9907, 4.0267)
  line L134 (88.9907, 4.0267) -> (88.9907, 3.0887)
  line L135 (88.9907, 3.0887) -> (88.8326, 3.0887)
  line L136 (88.8326, 3.0887) -> (88.8326, 3.192)
  spline S162 degree 2 poles (88.8326, 3.192) (88.7709, 3.1302) (88.6493, 3.0623) (88.5764, 3.0623) knots 0 0 0 1 2 2 2
  spline S163 degree 2 poles (88.5764, 3.0623) (88.4933, 3.0623) (88.3647, 3.1383) (88.3312, 3.2244) knots 0 0 0 1 2 2 2
  spline S164 degree 2 poles (88.3312, 3.2244) (88.2593, 3.1444) (88.1236, 3.0623) (88.0446, 3.0623) knots 0 0 0 1 2 2 2
  spline S165 degree 2 poles (88.0446, 3.0623) (87.9838, 3.0623) (87.8845, 3.0998) (87.848, 3.1424) knots 0 0 0 1 2 2 2
  spline S166 degree 2 poles (87.848, 3.1424) (87.8106, 3.1849) (87.769, 3.3125) (87.769, 3.4088) knots 0 0 0 1 2 2 2
  line L137 (87.769, 3.4088) -> (87.769, 4.0267)
  line L138 (87.769, 4.0267) -> (87.9271, 4.0267)
  spline S167 degree 2 poles (86.6497, 4.049) (86.7854, 4.049) (86.9759, 3.9922) (87.06, 3.9517) knots 0 0 0 1 2 2 2
  line L139 (87.06, 3.9517) -> (87.06, 3.743)
  line L140 (87.06, 3.743) -> (87.0478, 3.743)
  spline S168 degree 2 poles (87.0478, 3.743) (86.9657, 3.82) (86.7581, 3.9051) (86.6619, 3.9051) knots 0 0 0 1 2 2 2
  spline S169 degree 2 poles (86.6619, 3.9051) (86.5241, 3.9051) (86.3833, 3.7907) (86.3833, 3.6964) knots 0 0 0 1 2 2 2
  spline S170 degree 2 poles (86.3833, 3.6964) (86.3833, 3.6215) (86.4572, 3.5283) (86.5373, 3.505) knots 0 0 0 1 2 2 2
  spline S171 degree 2 poles (86.5373, 3.505) (86.595, 3.4888) (86.6912, 3.4665) (86.7632, 3.4483) knots 0 0 0 1 2 2 2
  spline S172 degree 2 poles (86.7632, 3.4483) (86.828, 3.4311) (86.9303, 3.3794) (86.9698, 3.3379) knots 0 0 0 1 2 2 2
  spline S173 degree 2 poles (86.9698, 3.3379) (87.0083, 3.2963) (87.0508, 3.1849) (87.0508, 3.112) knots 0 0 0 1 2 2 2
  spline S174 degree 2 poles (87.0508, 3.112) (87.0508, 2.96) (86.8138, 2.7544) (86.6305, 2.7544) knots 0 0 0 1 2 2 2
  spline S175 degree 2 poles (86.6305, 2.7544) (86.5251, 2.7544) (86.3387, 2.7959) (86.2587, 2.8354) knots 0 0 0 1 2 2 2
  line L141 (86.2587, 2.8354) -> (86.2587, 3.034)
  line L142 (86.2587, 3.034) -> (86.2709, 3.034)
  spline S176 degree 2 poles (86.2709, 3.034) (86.3306, 2.9793) (86.517, 2.8982) (86.6193, 2.8982) knots 0 0 0 1 2 2 2
  spline S177 degree 2 poles (86.6193, 2.8982) (86.7348, 2.8982) (86.8776, 3.0066) (86.8776, 3.0947) knots 0 0 0 1 2 2 2
  spline S178 degree 2 poles (86.8776, 3.0947) (86.8776, 3.1738) (86.7935, 3.268) (86.7145, 3.2892) knots 0 0 0 1 2 2 2
  spline S179 degree 2 poles (86.7145, 3.2892) (86.6619, 3.3034) (86.5089, 3.3399) (86.4583, 3.3551) knots 0 0 0 1 2 2 2
  spline S180 degree 2 poles (86.4583, 3.3551) (86.3296, 3.3946) (86.2101, 3.5536) (86.2101, 3.6701) knots 0 0 0 1 2 2 2
  spline S181 degree 2 poles (86.2101, 3.6701) (86.2101, 3.7441) (86.2698, 3.8859) (86.3235, 3.9355) knots 0 0 0 1 2 2 2
  spline S182 degree 2 poles (86.3235, 3.9355) (86.3833, 3.9902) (86.5352, 4.049) (86.6497, 4.049) knots 0 0 0 1 2 2 2
  spline S183 degree 2 poles (85.2822, 3.5577) (85.2822, 3.7947) (85.5101, 4.053) (85.7006, 4.053) knots 0 0 0 1 2 2 2
  spline S184 degree 2 poles (85.7006, 4.053) (85.8961, 4.053) (86.1199, 3.7866) (86.1199, 3.5577) knots 0 0 0 1 2 2 2
  spline S185 degree 2 poles (86.1199, 3.5577) (86.1199, 3.3227) (85.889, 3.0623) (85.7006, 3.0623) knots 0 0 0 1 2 2 2
  spline S186 degree 2 poles (85.7006, 3.0623) (85.5101, 3.0623) (85.2822, 3.3217) (85.2822, 3.5577) knots 0 0 0 1 2 2 2
  spline S187 degree 2 poles (85.4453, 3.5577) (85.4453, 3.3753) (85.578, 3.1981) (85.7006, 3.1981) knots 0 0 0 1 2 2 2
  spline S188 degree 2 poles (85.7006, 3.1981) (85.8231, 3.1981) (85.9568, 3.3753) (85.9568, 3.5577) knots 0 0 0 1 2 2 2
  spline S189 degree 2 poles (85.9568, 3.5577) (85.9568, 3.7349) (85.8231, 3.9173) (85.7006, 3.9173) knots 0 0 0 1 2 2 2
  spline S190 degree 2 poles (85.7006, 3.9173) (85.579, 3.9173) (85.4453, 3.738) (85.4453, 3.5577) knots 0 0 0 1 2 2 2
  spline S191 degree 2 poles (84.3341, 3.5425) (84.3341, 3.7724) (84.5569, 4.053) (84.7251, 4.053) knots 0 0 0 1 2 2 2
  spline S192 degree 2 poles (84.7251, 4.053) (84.801, 4.053) (84.9094, 4.0155) (84.9621, 3.9831) knots 0 0 0 1 2 2 2
  line L143 (84.9621, 3.9831) -> (84.9722, 4.0267)
  line L144 (84.9722, 4.0267) -> (85.1201, 4.0267)
  line L145 (85.1201, 4.0267) -> (85.1201, 2.721)
  line L146 (85.1201, 2.721) -> (84.9621, 2.721)
  line L147 (84.9621, 2.721) -> (84.9621, 3.1869)
  spline S193 degree 2 poles (84.9621, 3.1869) (84.9023, 3.1332) (84.7636, 3.0623) (84.6754, 3.0623) knots 0 0 0 1 2 2 2
  spline S194 degree 2 poles (84.6754, 3.0623) (84.5164, 3.0623) (84.3341, 3.3166) (84.3341, 3.5425) knots 0 0 0 1 2 2 2
  spline S195 degree 2 poles (84.4972, 3.5546) (84.4972, 3.3865) (84.5995, 3.2123) (84.7129, 3.2123) knots 0 0 0 1 2 2 2
  spline S196 degree 2 poles (84.7129, 3.2123) (84.7767, 3.2123) (84.9084, 3.273) (84.9621, 3.3196) knots 0 0 0 1 2 2 2
  line L148 (84.9621, 3.3196) -> (84.9621, 3.8575)
  spline S197 degree 2 poles (84.9621, 3.8575) (84.9023, 3.8869) (84.8102, 3.9112) (84.7555, 3.9112) knots 0 0 0 1 2 2 2
  spline S198 degree 2 poles (84.7555, 3.9112) (84.6349, 3.9112) (84.4972, 3.74) (84.4972, 3.5546) knots 0 0 0 1 2 2 2
  spline S199 degree 2 poles (83.7972, 4.0479) (83.8944, 4.0479) (84.0555, 3.9882) (84.1132, 3.9274) knots 0 0 0 1 2 2 2
  spline S200 degree 2 poles (84.1132, 3.9274) (84.171, 3.8676) (84.2348, 3.6833) (84.2348, 3.5597) knots 0 0 0 1 2 2 2
  spline S201 degree 2 poles (84.2348, 3.5597) (84.2348, 3.4361) (84.1689, 3.2558) (84.1132, 3.195) knots 0 0 0 1 2 2 2
  spline S202 degree 2 poles (84.1132, 3.195) (84.0575, 3.1332) (83.8924, 3.0674) (83.7972, 3.0674) knots 0 0 0 1 2 2 2
  spline S203 degree 2 poles (83.7972, 3.0674) (83.7202, 3.0674) (83.5764, 3.111) (83.5207, 3.1393) knots 0 0 0 1 2 2 2
  line L149 (83.5207, 3.1393) -> (83.5207, 3.3166)
  line L150 (83.5207, 3.3166) -> (83.5298, 3.3166)
  spline S204 degree 2 poles (83.5298, 3.3166) (83.547, 3.3024) (83.5997, 3.2659) (83.6371, 3.2467) knots 0 0 0 1 2 2 2
  spline S205 degree 2 poles (83.6371, 3.2467) (83.6706, 3.2305) (83.7597, 3.2052) (83.8002, 3.2052) knots 0 0 0 1 2 2 2
  spline S206 degree 2 poles (83.8002, 3.2052) (83.9228, 3.2052) (84.0717, 3.3905) (84.0717, 3.5597) knots 0 0 0 1 2 2 2
  spline S207 degree 2 poles (84.0717, 3.5597) (84.0717, 3.7248) (83.9279, 3.9102) (83.8002, 3.9102) knots 0 0 0 1 2 2 2
  spline S208 degree 2 poles (83.8002, 3.9102) (83.7232, 3.9102) (83.5835, 3.8464) (83.5298, 3.7967) knots 0 0 0 1 2 2 2
  line L151 (83.5298, 3.7967) -> (83.5207, 3.7967)
  line L152 (83.5207, 3.7967) -> (83.5207, 3.974)
  spline S209 degree 2 poles (83.5207, 3.974) (83.5439, 3.9851) (83.6149, 4.0165) (83.6432, 4.0236) knots 0 0 0 1 2 2 2
  spline S210 degree 2 poles (83.6432, 4.0236) (83.6837, 4.0358) (83.7476, 4.0479) (83.7972, 4.0479) knots 0 0 0 1 2 2 2
  line L153 (83.5409, 2.6197) -> (83.7324, 2.9377)
  line L154 (83.7324, 2.9377) -> (83.9228, 2.9377)
  line L155 (83.9228, 2.9377) -> (84.1142, 2.6197)
  line L156 (84.1142, 2.6197) -> (83.9805, 2.6197)
  line L157 (83.9805, 2.6197) -> (83.8256, 2.8344)
  line L158 (83.8256, 2.8344) -> (83.6706, 2.6197)
  line L159 (83.6706, 2.6197) -> (83.5409, 2.6197)
  line L160 (82.6475, 4.0267) -> (82.8055, 4.0267)
  line L161 (82.8055, 4.0267) -> (82.8055, 3.9234)
  spline S211 degree 2 poles (82.8055, 3.9234) (82.8784, 3.9872) (83.0091, 4.053) (83.0901, 4.053) knots 0 0 0 1 2 2 2
  spline S212 degree 2 poles (83.0901, 4.053) (83.1509, 4.053) (83.2593, 4.0125) (83.2988, 3.9689) knots 0 0 0 1 2 2 2
  spline S213 degree 2 poles (83.2988, 3.9689) (83.3393, 3.9254) (83.3839, 3.7927) (83.3839, 3.6975) knots 0 0 0 1 2 2 2
  line L162 (83.3839, 3.6975) -> (83.3839, 3.0887)
  line L163 (83.3839, 3.0887) -> (83.2259, 3.0887)
  line L164 (83.2259, 3.0887) -> (83.2259, 3.6235)
  spline S214 degree 2 poles (83.2259, 3.6235) (83.2259, 3.6985) (83.2147, 3.7967) (83.1955, 3.8332) knots 0 0 0 1 2 2 2
  spline S215 degree 2 poles (83.1955, 3.8332) (83.1762, 3.8697) (83.1104, 3.9031) (83.0486, 3.9031) knots 0 0 0 1 2 2 2
  spline S216 degree 2 poles (83.0486, 3.9031) (82.9909, 3.9031) (82.8602, 3.8373) (82.8055, 3.7896) knots 0 0 0 1 2 2 2
  line L165 (82.8055, 3.7896) -> (82.8055, 3.0887)
  line L166 (82.8055, 3.0887) -> (82.6475, 3.0887)
  line L167 (82.6475, 3.0887) -> (82.6475, 4.0267)
  line L168 (81.6416, 4.0267) -> (81.8493, 4.0267)
  line L169 (81.8493, 4.0267) -> (82.1977, 3.5739)
  line L170 (82.1977, 3.5739) -> (82.2605, 3.6347)
  line L171 (82.2605, 3.6347) -> (82.2605, 4.0267)
  line L172 (82.2605, 4.0267) -> (82.4185, 4.0267)
  line L173 (82.4185, 4.0267) -> (82.4185, 2.721)
  line L174 (82.4185, 2.721) -> (82.2605, 2.721)
  line L175 (82.2605, 2.721) -> (82.2605, 3.4847)
  line L176 (82.2605, 3.4847) -> (81.8898, 3.0887)
  line L177 (81.8898, 3.0887) -> (81.6933, 3.0887)
  line L178 (81.6933, 3.0887) -> (82.0782, 3.4807)
  line L179 (82.0782, 3.4807) -> (81.6416, 4.0267)
  point P0 (50, 15)
  dimension "d0" = 3
  dimension "d1" = 30
  dimension "d2" = 25
  constraints: 2 other
extrude "Vysunutí3" cut sketch "Náčrt3" against normal blind 0.2 contours L8 L9 L10 L11 L12 L13 L14 L15 L16 L17 | S0 S1 S2 S3 L18 L19 S4 S5 S6 L20 L21 S7 S8 | S13 S14 S15 S16 | S21 L23 L24 S22 S23 S24 S25 S26 S27 S28 S29 L25 L26 S30 S31 S32 S33 S34 S35 S36 | L27 L28 S37 S38 S39 L29 L30 L31 S40 S41 S42 L32 L33 L34 | L35 S43 S44 S45 S46 L36 L37 L38 S47 S48 S49 L39 L40 L41 L42 L43 S50 S51 S52 S53 S54 L44 L45 | S55 S56 S57 S58 L46 L47 S59 S60 S61 L48 L49 S62 S63 | S68 S69 S70 S71 S72 L51 L52 S73 S74 S75 S76 S77 L53 L54 S78 S79 | L55 L56 L57 L58 L59 L60 L61 L62 L63 L64 L65 L66 L67 | S80 S81 S82 S83 S84 S85 L68 S86 S87 S88 L69 L70 S89 S90 S91 L71 L72 L73 | L75 L76 S96 S97 S98 S99 S100 S101 S102 L77 L78 L79 | S107 S108 S109 S110 L81 L82 S111 S112 S113 L83 L84 S114 S115 | S120 S121 L86 L87 L88 L89 L90 S122 S123 | L92 L93 L94 L95 L96 L97 L98 L99 | L100 L101 L102 L103 L104 L105 L106 | S128 S129 S130 S131 S132 S133 L107 S134 S135 S136 L108 L109 S137 S138 S139 L110 L111 L112 | L114 L115 S144 S145 S146 S147 S148 S149 S150 L116 L117 L118 | L120 L121 L122 L123 | L124 L125 L126 L127 | L128 S155 S156 S157 S158 L129 L130 L131 S159 S160 S161 L132 L133 L134 L135 L136 S162 S163 S164 S165 S166 L137 L138 | S167 L139 L140 S168 S169 S170 S171 S172 S173 S174 S175 L141 L142 S176 S177 S178 S179 S180 S181 S182 | S183 S184 S185 S186 | S191 S192 L143 L144 L145 L146 L147 S193 S194 | S199 S200 S201 S202 S203 L149 L150 S204 S205 S206 S207 S208 L151 L152 S209 S210 | L153 L154 L155 L156 L157 L158 L159 | L160 L161 S211 S212 S213 L162 L163 L164 S214 S215 S216 L165 L166 L167 | L168 L169 L170 L171 L172 L173 L174 L175 L176 L177 L178 L179
chamfer "Zkosení1" distance 0.5 angle 45 3 edges at (-36.5, 1.5, -5.5) (-1.5, 1.5, -5.5) (33.5, 1.5, -5.5)
